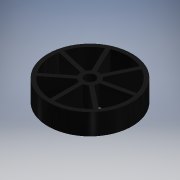
# Autodesk Inventor part: intake roller
Saved by Autodesk Inventor 2017 SP1 (Build 210196100, 196)
## iProperties
Created: 2018-01-19
Part Number: intake roller
Material: Rubber
Document SubType Name: Modeling
Designer: Ben
Appearance: Glossy - Black
Surface Area: 347.834 cm^2
Volume: 73.0662 cm^3
Mass: 67.9515 g
Density: 0.93 g/cm^3
Author: Ben
Autodesk Inventor part; units mm, degrees
ref_plane "YZ Plane" through (0, 0, 0) normal (1, 0, 0) x (0, 1, 0)
ref_plane "XZ Plane" through (0, 0, 0) normal (0, 1, 0) x (-1, 0, 0)
ref_plane "XY Plane" through (0, 0, 0) normal (0, 0, 1) x (1, 0, 0)
sketch "Sketch1" plane through (0, 0, 0) normal (0, 1, 0) x (-1, 0, 0)
  circle A0 centre (0, 0) radius 6.35
  circle A1 centre (0, 0) radius 50.8
  arc A2 (-17.8028, -42.456) -> (17.8028, -42.456) centre (0, 0) ccw
  line L0 (0, 0) -> (0, -50.8) construction
  arc A3 (-2.5641, -10.8126) -> (2.5641, -10.8126) centre (0, 0) ccw
  line L1 (17.8028, -42.456) -> (2.5641, -10.8126)
  line L2 (-2.5641, -10.8126) -> (-17.8028, -42.456)
  line L3 (6.855, -8.7463) -> (22.0936, -40.3896)
  arc A4 (22.0936, -40.3896) -> (44.2933, -12.5521) centre (0, 0) ccw
  line L4 (44.2933, -12.5521) -> (10.0523, -4.7369)
  arc A5 (6.855, -8.7463) -> (10.0523, -4.7369) centre (0, 0) ccw
  line L5 (11.1121, -0.0938) -> (45.353, -7.909)
  arc A6 (45.353, -7.909) -> (37.4301, 26.8038) centre (0, 0) ccw
  line L6 (37.4301, 26.8038) -> (9.971, 4.9059)
  arc A7 (11.1121, -0.0938) -> (9.971, 4.9059) centre (0, 0) ccw
  line L7 (7.0016, 8.6293) -> (34.4607, 30.5272)
  arc A8 (34.4607, 30.5272) -> (2.3812, 45.9759) centre (0, 0) ccw
  line L8 (2.3812, 45.9759) -> (2.3812, 10.8544)
  arc A9 (7.0016, 8.6293) -> (2.3812, 10.8544) centre (0, 0) ccw
  line L9 (-2.3813, 10.8544) -> (-2.3813, 45.9759)
  arc A10 (-2.3813, 45.9759) -> (-34.4607, 30.5272) centre (0, 0) ccw
  line L10 (-34.4607, 30.5272) -> (-7.0016, 8.6293)
  arc A11 (-2.3813, 10.8544) -> (-7.0016, 8.6293) centre (0, 0) ccw
  line L11 (-9.971, 4.9059) -> (-37.4301, 26.8038)
  arc A12 (-37.4301, 26.8038) -> (-45.353, -7.909) centre (0, 0) ccw
  line L12 (-45.353, -7.909) -> (-11.1121, -0.0938)
  arc A13 (-9.971, 4.9059) -> (-11.1121, -0.0938) centre (0, 0) ccw
  line L13 (-10.0523, -4.7369) -> (-44.2933, -12.5521)
  arc A14 (-44.2933, -12.5521) -> (-22.0936, -40.3896) centre (0, 0) ccw
  line L14 (-22.0936, -40.3896) -> (-6.855, -8.7463)
  arc A15 (-10.0523, -4.7369) -> (-6.855, -8.7463) centre (0, 0) ccw
  point P0 (0, -46.0375)
  point P1 (0, -11.1125)
  point P2 (35.9936, -28.7039)
  point P3 (8.6881, -6.9285)
  point P4 (44.8832, 10.2443)
  point P5 (10.8339, 2.4728)
  point P6 (19.9749, 41.4784)
  point P7 (4.8215, 10.012)
  point P8 (-19.9749, 41.4784)
  point P9 (-4.8215, 10.012)
  point P10 (-44.8832, 10.2443)
  point P11 (-10.8339, 2.4728)
  point P12 (-35.9936, -28.7039)
  point P13 (-8.6881, -6.9285)
  dimension "d1" = 101.6
  dimension "d0" = 12.7
  dimension "d4" = 4.7625
  dimension "d5" = 4.7625
  dimension "d8" = 360
  dimension "d10" = 4.7625
  constraints: 30 end point, 30 point on circle, 15 centre point, 10 coincident, 2 point on line, 1 parallel, 1 vertical, 1 vertical alignment, 87 other
  measures "d0" diameter of A0
  measures "d5" radial gap between concentric circles of A0 A3
  measures "d10" distance between parallel lines of L2 L14
extrude "Extrusion1" add sketch "Sketch1" along normal mid plane 25.4
equation "\"d5\" = d4"
equation "\"d10\" = d4"
body "Solid1"
